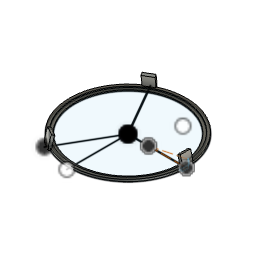
ikea-tertial-filter-mount v3 (Autodesk Fusion 360 design; units mm, degrees)
Autodesk Fusion 360 part; units mm, degrees
sketch "Sketch1" plane through (0, 0, 0) normal (0, 0, 1) x (1, 0, 0)
  circle A0 centre (0, 0) radius 85
  circle A1 centre (0, 0) radius 77
  circle A2 centre (0, 0) radius 81
  line L0 (87.0286, 7.5) -> (83.0286, 7.5)
  line L1 (83.0286, 7.5) -> (83.0286, -7.5)
  line L2 (83.0286, -7.5) -> (87.0286, -7.5)
  line L3 (87.0286, -7.5) -> (87.0286, 7.5)
  line L4 (87.0286, 7.5) -> (83.0286, -7.5) construction
  line L5 (83.0286, 7.5) -> (87.0286, -7.5) construction
  point P0 (85, 0)
  point P1 (85.0286, 0)
  dimension "d1" = 170
  dimension "d2" = 154
  dimension "d28" = 162
  dimension "d49" = 4
  dimension "d50" = 15
  constraint coincident A0.centre A1.centre
  constraint concentric A0 A1
  constraint coincident A0 P0
  constraint concentric A1 A2
  constraint horizontal L0
  constraint perpendicular L0 L1
  constraint parallel L0 L2
  constraint parallel L1 L3
  constraint coincident L4 P1
  constraint coincident L5 P1
  measures "d1" diameter of A0
  measures "d2" diameter of A1
  measures "d28" diameter of A2
  measures "d49" distance of L1.end L2.end
  measures "d50" distance of L0.end L1.end
sketch "Sketch7" plane through (0, 0, 0) normal (0, 0, 1) x (1, 0, 0)
  line L0 (89, 0) -> (0, 0)
  line L1 (0, 0) -> (-44.5, 77.0763)
  line L2 (-44.5, 77.0763) -> (0, 0)
  line L3 (-44.5, 77.0763) -> (0, 0)
  line L4 (0, 0) -> (89, 0)
  dimension "d9" = 89
  dimension "d10" = 120
  constraint coincident L0.end L1.start
  constraint horizontal L0
  measures "d9" distance of L0.end L1.end
  measures "d10" angle of L0 L1
sketch "Sketch10" plane through (0, 0, 0) normal (0, 0, 1) x (1, 0, 0)
  line L0 (0, -89) -> (0, 0)
  line L1 (0, 0) -> (-44.5, -77.0763)
  dimension "d11" = 89
  dimension "d12" = 30
  constraint coincident L0.end L1.start
  constraint vertical L0
  measures "d11" distance of L0.end L1.end
  measures "d12" angle of L0 L1
sketch "Sketch12" plane through (0, 0, 0) normal (0, 0, 1) x (1, 0, 0)
  point P0 (30, 0)
  point P1 (30, 50)
sketch "Sketch14" plane through (0, 0, 0) normal (0, 1, 0) x (1, 0, 0)
  arc A0 (87.6412, -12.1381) -> (88.9052, 0.1114) centre (30, 0) ccw
  line L0 (30, 0) -> (87.6412, -12.1381) construction
  line L1 (30, 0) -> (88.9052, 0.1114) construction
  dimension "d18" = 12
  measures "d18" angle of L0 L1
extrude "Extrude7" add sketch "Sketch1" along normal blind 1.5 contours A2 makes body 1
extrude "Extrude8" add sketch "Sketch1" along normal blind 3 contours A0 L0 L1 L2 picked at (-81.9532, -6.1322) bodies 1
revolve "Revolve3" add sketch "Sketch1" angle 20 about axis through (30, -10, 0) along (0, -1, 0) separate body contours A0 L0 L1 L2 | A0 L0 L2 L3 picked at (83.6857, 0) makes body 2
pattern_circular "C-Pattern2" count 3 over 360 about axis through (0, 0, 1.75) along (0, 0, 1) of bodies 2 makes body 3 at (-45.3369, 73.5258, 8.812) makes body 4 at (-45.5936, -73.9705, 4.4193)
combine "Combine1" operation add target body 1 tool bodies 4 3 2
